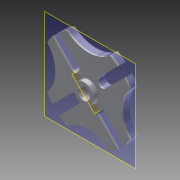
# Autodesk Inventor part: Geneva Driven
Saved by Autodesk Inventor 2018 (Build 220112000, 112)
## iProperties
Created: 2018-01-19
Part Number: Geneva Driven
Material: ABS Plastic
Document SubType Name: Modeling
Designer: Rus
Density: 1.06 g/cm^3
Appearance: Smooth - White
Mass: 106.579 g
Surface Area: 264.576 cm^2
Volume: 100.546 cm^3
Author: Rus
Autodesk Inventor part; units mm, degrees
ref_plane "YZ Plane" through (0, 0, 0) normal (1, 0, 0) x (0, 1, 0)
ref_plane "XZ Plane" through (0, 0, 0) normal (0, 1, 0) x (-1, 0, 0)
ref_plane "XY Plane" through (0, 0, 0) normal (0, 0, 1) x (1, 0, 0)
sketch "Sketch4" plane through (0, 0, 0) normal (0, 0, 1) x (1, 0, 0)
  line L0 (0, 0) -> (44.9009, -44.9017) construction
  line L1 (44.9009, -44.9017) -> (89.8017, 0) construction
  line L2 (89.8017, 0) -> (0, 0) construction
  circle A0 centre (0, 0) radius 63.5 construction
  line L3 (40.1856, -49.1667) -> (14.1078, -23.0884)
  line L4 (23.0881, -14.1082) -> (49.166, -40.1866)
  arc A1 (23.0881, -14.1082) -> (14.1078, -23.0884) centre (18.5979, -18.5983) ccw
  arc A2 (56.3508, 29.2718) -> (56.3508, -29.2718) centre (89.8017, 0) ccw
  arc A3 (49.166, -40.1866) -> (56.3508, -29.2718) centre (0, 0) ccw
  arc A4 (56.3508, 29.2718) -> (49.166, 40.1866) centre (0, 0) ccw
  line L5 (49.166, 40.1866) -> (56.3508, 29.2718) construction
  line L6 (56.3508, -29.2718) -> (49.166, -40.1866) construction
  line L7 (0, 0) -> (44.9017, 44.9009) construction
  line L8 (44.9017, 44.9009) -> (0, 89.8017) construction
  line L9 (0, 89.8017) -> (0, 0) construction
  circle A5 centre (0, 0) radius 63.5 construction
  line L10 (49.166, 40.1866) -> (23.0884, 14.1078)
  line L11 (14.1082, 23.0881) -> (40.1866, 49.166)
  arc A6 (14.1082, 23.0881) -> (23.0884, 14.1078) centre (18.5983, 18.5979) ccw
  arc A7 (-29.2718, 56.3508) -> (29.2718, 56.3508) centre (0, 89.8017) ccw
  arc A8 (40.1866, 49.166) -> (29.2718, 56.3508) centre (0, 0) ccw
  arc A9 (-29.2718, 56.3508) -> (-40.1856, 49.1667) centre (0, 0) ccw
  line L12 (-40.1856, 49.1667) -> (-29.2718, 56.3508) construction
  line L13 (29.2718, 56.3508) -> (40.1866, 49.166) construction
  line L14 (0, 0) -> (-44.9008, 44.9017) construction
  line L15 (-44.9008, 44.9017) -> (-89.8017, 0) construction
  line L16 (-89.8017, 0) -> (0, 0) construction
  circle A10 centre (0, 0) radius 63.5 construction
  line L17 (-40.1856, 49.1667) -> (-14.1078, 23.0884)
  line L18 (-23.0881, 14.1082) -> (-49.166, 40.1866)
  arc A11 (-23.0881, 14.1082) -> (-14.1078, 23.0884) centre (-18.5979, 18.5983) ccw
  arc A12 (-56.3508, -29.2718) -> (-56.3508, 29.2718) centre (-89.8017, 0) ccw
  arc A13 (-49.166, 40.1866) -> (-56.3508, 29.2718) centre (0, 0) ccw
  arc A14 (-56.3508, -29.2718) -> (-49.1667, -40.1856) centre (0, 0) ccw
  line L19 (-49.1667, -40.1856) -> (-56.3508, -29.2718) construction
  line L20 (-56.3508, 29.2718) -> (-49.166, 40.1866) construction
  line L21 (0, 0) -> (-44.9017, -44.9008) construction
  line L22 (-44.9017, -44.9008) -> (0, -89.8017) construction
  line L23 (0, -89.8017) -> (0, 0) construction
  circle A15 centre (0, 0) radius 63.5 construction
  line L24 (-49.1667, -40.1856) -> (-23.0884, -14.1078)
  line L25 (-14.1082, -23.0881) -> (-40.1866, -49.166)
  arc A16 (-14.1082, -23.0881) -> (-23.0884, -14.1078) centre (-18.5983, -18.5979) ccw
  arc A17 (29.2718, -56.3508) -> (-29.2718, -56.3508) centre (0, -89.8017) ccw
  arc A18 (-40.1866, -49.166) -> (-29.2718, -56.3508) centre (0, 0) ccw
  arc A19 (29.2718, -56.3508) -> (40.1856, -49.1667) centre (0, 0) ccw
  line L26 (40.1856, -49.1667) -> (29.2718, -56.3508) construction
  line L27 (-29.2718, -56.3508) -> (-40.1866, -49.166) construction
  dimension "d22" = 89.8017
  dimension "d23" = 63.5
  dimension "d27" = 12.7
  dimension "d28" = 37.1983
  dimension "d29" = 44.45
  constraints: 56 end point, 56 point on circle, 20 centre point, 16 coincident, 4 point on line, 2 equal length, 2 parallel, 2 tangent, 1 concentric, 1 horizontal
  measures "d22" distance of L1.end L0.start
  measures "d23" distance of L0.end L1.end
  measures "d27" distance between parallel lines of L3 L4
  measures "d28" distance of A1.centre L0.end
  measures "d29" radius of A2
extrude "Extrusion3" add sketch "Sketch4" along normal blind 16.9333
ref_plane "Work Plane1" through (0, 0, 8.4667) normal (0, 0, -1) x (-1, 0, 0)
sketch "Sketch19" plane through (0, 0, 16.9333) normal (0, 0, 1) x (1, 0, 0)
  circle A0 centre (0, 0) radius 8.4667
  dimension "d93" = 16.9333
  constraints: 1 centre point, 1 coincident
  measures "d93" diameter of A0
extrude "Extrusion15" cut sketch "Sketch19" against normal through all
ref_plane "Work Plane5" through (14.1078, -14.1081, 0) normal (0.7071, 0.7071, 0) x (-0.7071, 0.7071, 0)
sketch "Sketch20" plane through (14.1078, -14.1081, 0) normal (0.7071, 0.7071, 0) x (-0.7071, 0.7071, 0)
  line L0 (-6.35, 0) -> (-6.35, 16.9333) projected
  line L1 (-6.35, 0) -> (-6.35, 16.9333)
  line L2 (-6.35, 16.9333) -> (-82.55, 16.9333)
  line L3 (-40.5924, 16.9333) -> (0.8046, 16.9333) projected
  line L4 (-82.55, 16.9333) -> (-82.55, 10.5833)
  line L5 (-6.35, 0) -> (-43.23, 0) projected
  line L6 (-82.55, 0) -> (-6.35, 0) construction
  line L7 (19.9517, 0) -> (19.9517, 76.2)
  line L8 (-6.35, 16.9333) -> (6.35, 16.9333)
  line L9 (6.35, 16.9333) -> (6.35, 0)
  line L10 (6.35, 0) -> (-6.35, 0)
  line L11 (-82.55, 16.9333) -> (-82.55, 10.5833)
  line L12 (-82.55, 10.5833) -> (-6.35, 10.5833)
  line L13 (-6.35, 10.5833) -> (6.35, 10.5833)
  line L14 (-82.55, 10.5833) -> (-82.55, 0) construction
  dimension "d96" = 76.2
  dimension "d97" = 76.2
  dimension "d98" = 12.7
  dimension "d99" = 6.35
  constraints: 24 end point, 5 point on line, 4 perpendicular, 3 collinear, 1 vertical
  measures "d96" distance of L0.end L2.end
  measures "d97" distance of L7.start L7.end
  measures "d98" distance of L0.end L8.end
  measures "d99" distance of L2.end L4.end
revolve "Revolution3" cut sketch "Sketch20" angle 360 about axis through (0, 0, 0) along (0, 0, 1) contours L12 L4 L2 L0 | L0 L3 L8 L9 L13
body "Solid2"
